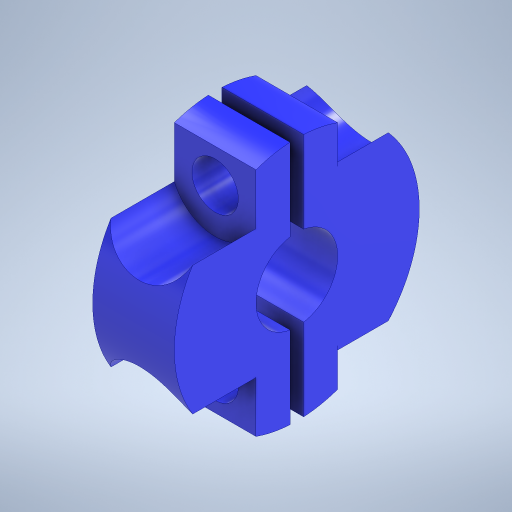
# Autodesk Inventor part: setcolor-6-18-3d
Saved by Autodesk Inventor 2024.1 (Build 281209000, 209)
## iProperties
Created: 2023-10-12
Part Number: setcolor-6-18-3d
Material: ABS プラスチック
Document SubType Name: Modeling
Designer: haruy
Density: 1.06 g/cm^3
Appearance: 青 - 壁塗料 - 光沢
Author: haruy
Autodesk Inventor part; units mm, degrees
ref_plane "YZ Plane" through (0, 0, 0) normal (1, 0, 0) x (0, 1, 0)
sketch "スケッチ1" plane through (0, 0, 0) normal (1, 0, 0) x (0, 1, 0)
  circle A0 centre (0, 0) radius 3
  circle A1 centre (0, 0) radius 9
  line L0 (-8.9861, 0.5) -> (8.9861, 0.5)
  line L1 (0, 0) -> (9, 0)
  line L2 (-8.9861, -0.5) -> (8.9861, -0.5)
  line L3 (0, 0) -> (0, -9)
  line L4 (8.4853, -3) -> (-8.4853, -3)
  point P0 (-2.958, 0.5)
  point P1 (2.958, 0.5)
  point P2 (-2.958, -0.5)
  point P3 (2.958, -0.5)
  dimension "d0" = 6
  dimension "d1" = 18
  dimension "d2" = 0.5
  dimension "d9" = 2.5
  constraints: 10 end point, 6 point on circle, 3 coincident, 3 horizontal, 2 centre point, 2 symmetric about line, 1 vertical
  measures "d0" diameter of A0
  measures "d1" diameter of A1
  measures "d2" distance from line of L0 point (0, 0)
  measures "d9" distance between parallel lines of L4 L2
extrude "押し出し1" add sketch "スケッチ1" along normal mid plane 6 contours A0 L0 A1 | L2 A1 L4 A0 | L4 A1 L2 A0 | L4 A1 L3 | L3 A1 L4
ref_plane "作業平面1" through (0, 0, -9) normal (0, 0, 1) x (1, 0, 0)
sketch "スケッチ2" plane through (0, 0, -9) normal (0, 0, 1) x (1, 0, 0)
  line L0 (-3, 8.9861) -> (3, 8.9861) projected
  line L1 (0, 0) -> (-3, 0)
  line L2 (-3, 8.9861) -> (-3, -8.9861) projected
  circle A0 centre (0, 5.9861) radius 1.7
  circle A1 centre (0, -5.9861) radius 1.7
  circle A2 centre (0, 5.9861) radius 3
  circle A3 centre (0, -5.9861) radius 3
  line L3 (3, -2.958) -> (3, -8.9861) projected
  line L4 (3, -5.9861) -> (3, -8.9861)
  line L5 (3, -8.9861) -> (0, -8.9861)
  line L6 (-3, -8.9861) -> (3, -8.9861) projected
  line L7 (0, -5.9861) -> (0, 5.9861)
  line L8 (-3, -2.958) -> (-3, -8.9861)
  line L9 (-3, -8.9861) -> (0, -8.9861)
  line L10 (-3, -8.9861) -> (-3, 8.9861)
  line L11 (3, 2.958) -> (3, 8.9861)
  line L12 (3, 8.9861) -> (0, 8.9861)
  line L13 (-3, 8.9861) -> (3, 8.9861)
  point P0 (-3, -5.9861)
  point P1 (3, 5.9861)
  point P2 (0, 8.9861)
  point P3 (-3, 5.9861)
  dimension "d11" = 6
  dimension "d5" = 3
  dimension "d6" = 3.4
  dimension "d10" = 6
  constraints: 20 end point, 7 symmetric about line, 3 centre point, 3 coincident, 2 midpoint, 2 vertical, 1 collinear, 4 other
  measures "d5" distance from line of L0 point (0, 5.986)
  measures "d6" diameter of A0
  measures "d10" diameter of A2
extrude "押し出し2" cut sketch "スケッチ2" along normal through all contours A0 | A1
extrude "押し出し3" cut sketch "スケッチ2" along normal blind 6 contours L0 A2 L2 | L0 L11 A2 | A2 | A3 | A3 L6 L2 | L3 L5 A3
ref_plane "作業平面2" through (0, 0, 9) normal (0, 0, -1) x (-1, 0, 0)
sketch "スケッチ3" plane through (0, 0, 9) normal (0, 0, -1) x (-1, 0, 0)
  line L0 (-3, 8.9861) -> (3, 8.9861)
  line L1 (0, 0) -> (-3, 0)
  line L2 (-3, 8.9861) -> (-3, -8.9861)
  circle A0 centre (0, 5.9861) radius 1.7
  circle A1 centre (0, -5.9861) radius 1.7
  circle A2 centre (0, 5.9861) radius 2.5
  circle A3 centre (0, -5.9861) radius 2.5
  circle A4 centre (0, 5.9861) radius 3.25
  circle A5 centre (0, -5.9861) radius 3.25
  line L3 (3, -8.9861) -> (-3, -8.9861) projected
  line L4 (3, -4.7361) -> (3, -8.9861)
  line L5 (3, -8.9861) -> (-3, -8.9861)
  line L6 (-3, -8.9861) -> (-3, -4.7361)
  line L7 (-3, -8.9861) -> (-3, 8.9861)
  line L8 (3, 8.9861) -> (-3, 8.9861)
  line L9 (3, 4.7361) -> (3, 8.9861)
  point P0 (0, 0)
  point P1 (3, 7.2361)
  point P2 (1.25, 8.9861)
  point P3 (-3, 7.2361)
  point P4 (-1.25, 8.9861)
  point P5 (-1.25, -8.9861)
  point P6 (-3, -7.2361)
  point P7 (3, -7.2361)
  point P8 (1.25, -8.9861)
  dimension "d14" = 3
  dimension "d15" = 3.4
  dimension "d16" = 5
  dimension "d17" = 5
  dimension "d18" = 6.5
  constraints: 18 end point, 6 centre point, 6 symmetric about line, 4 coincident, 2 point on circle, 1 midpoint, 1 perpendicular, 1 point on line, 1 vertical, 2 other
  measures "d14" distance from line of L0 point (0, 5.986)
  measures "d15" diameter of A0
  measures "d16" diameter of A2
  measures "d17" diameter of A3
  measures "d18" diameter of A4
extrude "押し出し4" cut sketch "スケッチ3" along normal blind 6 contours A5 L4 L3 L2 | L2 A5 | L0 A4 L2 | A4 L0 | L0 A4 L9 L2 | L2 A4 | L0 L9 A4 | A4 L9 | A5 L3 L2 | A5 L4 | L3 A5 | L4 L3 A5 | A2 | A3
